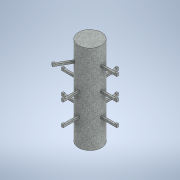
# Autodesk Inventor part: Central Coral
Saved by Autodesk Inventor 2021 (Build 250183000, 183)
## iProperties
Created: 2021-01-26
Part Number: Central Coral
Material: Generic
Document SubType Name: Modeling
Designer: aidan
Density: 1 g/cm^3
Appearance: Exposed Aggregate - Warm Gray
Author: aidan
Autodesk Inventor part; units mm, degrees
ref_plane "YZ Plane" through (0, 0, 0) normal (1, 0, 0) x (0, 1, 0)
ref_plane "XZ Plane" through (0, 0, 0) normal (0, 1, 0) x (-1, 0, 0)
ref_plane "XY Plane" through (0, 0, 0) normal (0, 0, 1) x (1, 0, 0)
sketch "Sketch1" plane through (0, 0, 0) normal (0, 1, 0) x (-1, 0, 0)
  line L0 (223.1291, -223.1291) -> (81.6709, -304.8)
  line L1 (81.6709, -304.8) -> (-81.6709, -304.8)
  line L2 (-81.6709, -304.8) -> (-223.1291, -223.1291)
  line L3 (-223.1291, -223.1291) -> (-304.8, -81.6709)
  line L4 (-304.8, -81.6709) -> (-304.8, 81.6709)
  line L5 (-304.8, 81.6709) -> (-223.1291, 223.1291)
  line L6 (-223.1291, 223.1291) -> (-81.6709, 304.8)
  line L7 (-81.6709, 304.8) -> (81.6709, 304.8)
  line L8 (81.6709, 304.8) -> (223.1291, 223.1291)
  line L9 (223.1291, 223.1291) -> (304.8, 81.6709)
  line L10 (304.8, 81.6709) -> (304.8, -81.6709)
  line L11 (304.8, -81.6709) -> (223.1291, -223.1291)
  point P0 (0, 0)
  point P1 (0, 0)
  dimension "d4" = 609.6
  constraints: 24 end point, 1 coincident, 1 vertical, 25 other
  measures "d4" distance between parallel lines of L4 L10
extrude "Extrusion1" add sketch "Sketch1" along normal blind 2438.4
sketch "Sketch2" plane through (304.8, 0, 81.6709) normal (1, 0, 0) x (0, 0, -1)
  line L0 (56.2709, 1981.2) -> (107.0709, 1981.2)
  line L1 (107.0709, 1981.2) -> (107.0709, 1930.4)
  line L2 (107.0709, 1930.4) -> (56.2709, 1930.4)
  line L3 (56.2709, 1930.4) -> (56.2709, 1981.2)
  line L4 (0, 2438.4) -> (163.3418, 2438.4) projected
  line L5 (163.3418, 2438.4) -> (0, 2438.4) projected
  line L6 (81.6709, 2438.4) -> (81.6709, 0) construction
  dimension "d5" = 457.2
  dimension "d6" = 50.8
  constraints: 10 end point, 2 parallel, 2 perpendicular, 1 horizontal, 1 midpoint, 1 vertical, 1 other
  measures "d5" distance between parallel lines of L4 L0
  measures "d6" distance of L0.start L0.end
extrude "Extrusion2" add sketch "Sketch2" along normal blind 457.2
sketch "Sketch3" plane through (304.8, 1981.2, 25.4) normal (0, 1, 0) x (1, 0, 0)
  line L0 (457.2, 0) -> (457.2, 50.8) projected
  line L1 (457.2, 0) -> (406.4, 0)
  line L2 (406.4, 0) -> (406.4, 50.8)
  line L3 (406.4, 50.8) -> (457.2, 50.8)
  line L4 (457.2, 50.8) -> (457.2, 0)
  point P0 (-304.8, 25.4)
  constraints: 8 end point, 2 parallel, 2 perpendicular, 1 horizontal
extrude "Extrusion3" add sketch "Sketch3" along normal blind 25.4
pattern_linear "Rectangular Pattern1" count 3 spacing 609.6 along (0, -1, 0) of "Extrusion3", "Extrusion2"
pattern_circular "Circular Pattern1" count 3 over 360 about axis through (0, 2438.4, 0) along (0, 1, 0) of "Extrusion2", "Extrusion3"
pattern_circular "Circular Pattern2" count 4 over 360 about axis through (0, 2438.4, 0) along (0, 1, 0) of "Extrusion3", "Extrusion2", "Rectangular Pattern1"
sketch "Sketch4" plane through (0, 2438.4, 0) normal (0, 1, 0) x (1, 0, 0)
  line L0 (81.6709, 304.8) -> (-81.6709, 304.8)
  line L1 (-81.6709, 304.8) -> (-81.6709, 762)
  line L2 (-81.6709, 762) -> (81.6709, 762)
  line L3 (81.6709, 762) -> (81.6709, 304.8)
  line L4 (25.4, 762) -> (-25.4, 762) projected
  point P0 (0, 0)
  constraints: 8 end point, 2 parallel, 1 collinear, 1 horizontal, 1 perpendicular
extrude "Extrusion4" cut sketch "Sketch4" against normal blind 508
pattern_circular "Circular Pattern3" count 3 over 180 about axis through (0, 2438.4, 0) along (0, 1, 0) of "Extrusion4"
sketch "Sketch5" plane through (0, 2438.4, 0) normal (0, 1, 0) x (1, 0, 0)
  line L0 (-81.6709, 304.8) -> (-223.1291, 223.1291) projected
  circle A0 centre (0, 0) radius 315.5522
  constraints: 1 coincident, 3 other
extrude "Extrusion5" add sketch "Sketch5" against normal blind 2438.4 contours A0 L0 picked at (-138.223, 29.6465)
body "Solid1"
